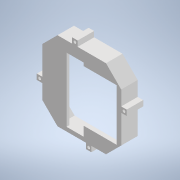
# Autodesk Inventor part: Низ
Saved by Autodesk Inventor 2021.2 (Build 252289000, 289)
## iProperties
Created: 2021-11-01
Part Number: Низ
Material: Типовые
Document SubType Name: Modeling
Designer: Kolan
Density: 1 g/cm^3
Appearance: По умолчанию
Author: Kolan
Autodesk Inventor part; units mm, degrees
ref_plane "YZ Plane" through (0, 0, 0) normal (1, 0, 0) x (0, 1, 0)
ref_plane "XZ Plane" through (0, 0, 0) normal (0, 1, 0) x (-1, 0, 0)
ref_plane "XY Plane" through (0, 0, 0) normal (0, 0, 1) x (1, 0, 0)
sketch "Эскиз1" plane through (0, 0, 0) normal (0, 0, 1) x (1, 0, 0)
  line L0 (0, 34.036) -> (-10.16, 44.196) construction
  line L1 (0, 0) -> (0, 34.036) construction
  line L2 (-10.16, -10.16) -> (0, 0) construction
  line L3 (-44.196, -10.16) -> (-10.16, -10.16) construction
  line L4 (-54.356, 0) -> (-44.196, -10.16) construction
  line L5 (-54.356, 34.036) -> (-54.356, 0) construction
  line L6 (-44.196, 44.196) -> (-54.356, 34.036) construction
  line L7 (-10.16, 44.196) -> (-44.196, 44.196) construction
  line L8 (1.5, -0.6213) -> (1.5, 34.6573)
  line L9 (1.5, 34.6573) -> (-9.5387, 45.696)
  line L10 (-9.5387, 45.696) -> (-44.8173, 45.696)
  line L11 (-44.8173, 45.696) -> (-55.856, 34.6573)
  line L12 (-55.856, 34.6573) -> (-55.856, -0.6213)
  line L13 (-55.856, -0.6213) -> (-44.8173, -11.66)
  line L14 (-44.8173, -11.66) -> (-9.5387, -11.66)
  line L15 (-9.5387, -11.66) -> (1.5, -0.6213)
  line L16 (-2.7356, -0.7983) -> (-25.2842, -0.7983) construction
  line L17 (-2.7356, 34.7503) -> (-2.7356, -0.7983) construction
  line L18 (-25.2842, 34.7503) -> (-2.7356, 34.7503) construction
  line L19 (-25.2842, -0.7983) -> (-25.2842, 34.7503) construction
  line L20 (-35.7877, 37.522) -> (-26.3913, 37.522) construction
  line L21 (-35.7877, -8.198) -> (-26.3913, -8.198) construction
  line L22 (-26.3913, -0.578) -> (-26.3913, -5.658) construction
  line L23 (-37.7413, -0.578) -> (-37.7413, -5.658) construction
  line L24 (-1.7356, -1.7983) -> (-26.2842, -1.7983)
  line L25 (-26.2842, -1.7983) -> (-26.2842, 35.7503)
  line L26 (-26.2842, 35.7503) -> (-1.7356, 35.7503)
  line L27 (-1.7356, 35.7503) -> (-1.7356, -1.7983)
  line L28 (-26.3913, 37.522) -> (-37.7413, 37.522) construction
  line L29 (-37.7413, 37.522) -> (-37.7413, -8.198) construction
  line L30 (-37.7413, -8.198) -> (-26.3913, -8.198) construction
  line L31 (-26.3913, -8.198) -> (-26.3913, 37.522) construction
  line L32 (-38.2413, 38.022) -> (-25.8913, 38.022)
  line L33 (-25.8913, 38.022) -> (-25.8913, -8.698)
  line L34 (-25.8913, -8.698) -> (-38.2413, -8.698)
  line L35 (-38.2413, -8.698) -> (-38.2413, 38.022)
  point P0 (-25.8913, -1.7983)
  point P1 (-25.8913, 35.7503)
  dimension "d0" = 1.5
  dimension "d1" = 1
  dimension "d2" = 0.5
  constraints: 40 end point, 4 parallel, 2 perpendicular, 1 horizontal, 1 point on line, 13 other
  measures "d0" distance between parallel lines of L2 L15
  measures "d1" distance between parallel lines of L17 L27
  measures "d2" distance between parallel lines of L28 L32
extrude "Выдавливание1" add sketch "Эскиз1" along normal blind 2
sketch "Эскиз2" plane through (0, 0, 0) normal (0, 0, -1) x (-1, 0, 0)
  line L0 (-1.5, 34.6573) -> (9.5387, 45.696) construction
  line L1 (-1.5, -0.6213) -> (-1.5, 34.6573) construction
  line L2 (9.5387, -11.66) -> (-1.5, -0.6213) construction
  line L3 (44.8173, -11.66) -> (9.5387, -11.66) construction
  line L4 (55.856, -0.6213) -> (44.8173, -11.66) construction
  line L5 (55.856, 34.6573) -> (55.856, -0.6213) construction
  line L6 (44.8173, 45.696) -> (55.856, 34.6573) construction
  line L7 (9.5387, 45.696) -> (44.8173, 45.696) construction
  line L8 (1.7356, 35.7503) -> (1.7356, -1.7983) construction
  line L9 (25.8913, 35.7503) -> (1.7356, 35.7503) construction
  line L10 (25.8913, 38.022) -> (25.8913, 35.7503) construction
  line L11 (38.2413, 38.022) -> (25.8913, 38.022) construction
  line L12 (38.2413, -8.698) -> (38.2413, 38.022) construction
  line L13 (25.8913, -8.698) -> (38.2413, -8.698) construction
  line L14 (25.8913, -1.7983) -> (25.8913, -8.698) construction
  line L15 (1.7356, -1.7983) -> (25.8913, -1.7983) construction
  line L16 (-0.5, 34.2431) -> (9.9529, 44.696)
  line L17 (9.9529, 44.696) -> (44.4031, 44.696)
  line L18 (44.4031, 44.696) -> (54.856, 34.2431)
  line L19 (54.856, 34.2431) -> (54.856, -0.2071)
  line L20 (54.856, -0.2071) -> (44.4031, -10.66)
  line L21 (44.4031, -10.66) -> (9.9529, -10.66)
  line L22 (9.9529, -10.66) -> (-0.5, -0.2071)
  line L23 (-0.5, -0.2071) -> (-0.5, 34.2431)
  line L24 (-1.5, 34.6573) -> (9.5387, 45.696)
  line L25 (9.5387, 45.696) -> (44.8173, 45.696)
  line L26 (44.8173, 45.696) -> (55.856, 34.6573)
  line L27 (55.856, 34.6573) -> (55.856, -0.6213)
  line L28 (55.856, -0.6213) -> (44.8173, -11.66)
  line L29 (44.8173, -11.66) -> (9.5387, -11.66)
  line L30 (9.5387, -11.66) -> (-1.5, -0.6213)
  line L31 (-1.5, -0.6213) -> (-1.5, 34.6573)
  point P0 (0, 0)
  dimension "d0" = 1.5
  dimension "d5" = 1
  dimension "d6" = 1
  constraints: 32 end point, 14 other
  measures "d5" distance between parallel lines of L1 L23
  measures "d6" distance between parallel lines of L23 L31
extrude "Выдавливание2" add sketch "Эскиз2" along normal blind 10
sketch "Эскиз3" plane through (0, 0, 2) normal (0, 0, 1) x (1, 0, 0)
  line L0 (-44.8173, -11.66) -> (-9.5387, -11.66) construction
  line L1 (-9.5387, 45.696) -> (-44.8173, 45.696) construction
  line L2 (-55.856, 34.6573) -> (-55.856, -0.6213) construction
  line L3 (1.5, -0.6213) -> (1.5, 34.6573) construction
  line L4 (-20.178, -11.66) -> (-24.178, -11.66)
  line L5 (-24.178, -11.66) -> (-24.178, -15.66)
  line L6 (-24.178, -15.66) -> (-20.178, -15.66)
  line L7 (-20.178, -15.66) -> (-20.178, -11.66)
  line L8 (-30.178, 45.696) -> (-34.178, 45.696)
  line L9 (-34.178, 45.696) -> (-34.178, 49.696)
  line L10 (-34.178, 49.696) -> (-30.178, 49.696)
  line L11 (-30.178, 49.696) -> (-30.178, 45.696)
  line L12 (1.5, 24.018) -> (5.5, 24.018)
  line L13 (5.5, 24.018) -> (5.5, 20.018)
  line L14 (5.5, 20.018) -> (1.5, 20.018)
  line L15 (1.5, 20.018) -> (1.5, 24.018)
  line L16 (-55.856, 10.018) -> (-59.856, 10.018)
  line L17 (-59.856, 10.018) -> (-59.856, 14.018)
  line L18 (-59.856, 14.018) -> (-55.856, 14.018)
  line L19 (-55.856, 14.018) -> (-55.856, 10.018)
  point P0 (0, 0)
  point P1 (-27.178, -11.66)
  point P2 (1.5, 17.018)
  point P3 (-55.856, 17.018)
  point P4 (-27.178, 45.696)
  dimension "d9" = 4
  dimension "d10" = 4
  dimension "d11" = 3
  dimension "d12" = 4
  dimension "d13" = 4
  dimension "d14" = 4
  dimension "d15" = 4
  dimension "d16" = 4
  dimension "d17" = 4
  dimension "d18" = 3
  dimension "d19" = 3
  dimension "d20" = 3
  constraints: 32 end point, 8 parallel, 4 horizontal, 4 midpoint, 4 perpendicular, 4 point on line
  measures "d9" distance of L6.end L5.end
  measures "d10" distance of L5.end L4.end
  measures "d11" distance from line of point (-27.178, -11.66) L5
  measures "d12" distance of L9.end L10.end
  measures "d13" distance of L8.end L9.end
  measures "d14" distance of L13.end L14.end
  measures "d15" distance of L12.end L13.end
  measures "d16" distance of L17.end L18.end
  measures "d17" distance of L16.end L17.end
  measures "d18" distance from line of point (-55.856, 17.018) L18
  measures "d19" distance from line of point (1.5, 17.018) L14
  measures "d20" distance from line of L11 point (-27.178, 45.696)
extrude "Выдавливание3" add sketch "Эскиз3" against normal up to surface (12 mm away)
sketch "Эскиз4" plane through (0, 0, -10) normal (0, 0, -1) x (-1, 0, 0)
  circle A0 centre (-3.5, 22.018) radius 1.5 construction
  circle A1 centre (32.178, 47.696) radius 1.5 construction
  circle A2 centre (57.856, 12.018) radius 1.5 construction
  circle A3 centre (22.178, -13.66) radius 1.5 construction
  circle A4 centre (22.178, -13.66) radius 1
  circle A5 centre (57.856, 12.018) radius 1
  circle A6 centre (32.178, 47.696) radius 1
  circle A7 centre (-3.5, 22.018) radius 1
  point P0 (0, 0)
  dimension "d23" = 2
  dimension "d24" = 2
  dimension "d25" = 2
  dimension "d27" = 2
  constraints: 4 centre point, 4 coincident
  measures "d23" diameter of A4
  measures "d24" diameter of A5
  measures "d25" diameter of A6
  measures "d27" diameter of A7
extrude "Выдавливание4" cut sketch "Эскиз4" against normal through all
